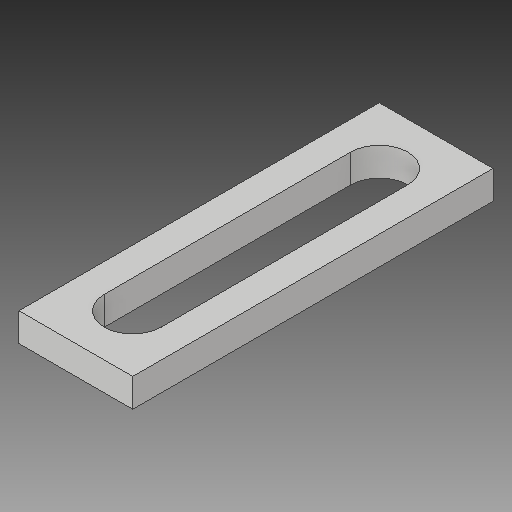
# Autodesk Inventor part: Marque
Saved by Autodesk Inventor 2017 (Build 210142000, 142)
## iProperties
Created: 2019-03-08
Part Number: Marque
Material: Generic
Document SubType Name: Modeling
Designer: Mitch
Density: 1 g/cm^3
Appearance: Default
Mass: 208.724 g
Surface Area: 425.806 cm^2
Volume: 208.724 cm^3
Author: Mitch
Autodesk Inventor part; units mm, degrees
ref_plane "YZ Plane" through (0, 0, 0) normal (1, 0, 0) x (0, 1, 0)
ref_plane "XZ Plane" through (0, 0, 0) normal (0, 1, 0) x (-1, 0, 0)
ref_plane "XY Plane" through (0, 0, 0) normal (0, 0, 1) x (1, 0, 0)
sketch "Sketch1" plane through (0, 0, 0) normal (0, 1, 0) x (-1, 0, 0)
  line L0 (0, 0) -> (76.2, 0)
  line L1 (76.2, 0) -> (76.2, -241.3)
  line L2 (76.2, -241.3) -> (0, -241.3)
  line L3 (0, -241.3) -> (0, 0)
  dimension "d0" = 76.2
  dimension "d1" = 241.3
  constraints: 8 end point, 2 parallel, 1 horizontal, 1 perpendicular
  measures "d0" distance of L1.end L2.end
  measures "d1" distance of L0.end L1.end
extrude "Extrusion1" add sketch "Sketch1" along normal blind 19.05
sketch "Sketch3" plane through (0, 19.05, 0) normal (0, 1, 0) x (1, 0, 0)
  line L0 (-76.2, 0) -> (0, 0) projected
  line L1 (0, 0) -> (0, 241.3) projected
  line L2 (0, 241.3) -> (-76.2, 241.3) projected
  line L3 (-76.2, 241.3) -> (-76.2, 0) projected
  line L4 (-38.1, 19.05) -> (-38.1, 19.05)
  line L5 (-19.05, 38.1) -> (-19.05, 203.2)
  line L6 (-38.1, 222.25) -> (-38.1, 222.25)
  line L7 (-57.15, 203.2) -> (-57.15, 38.1)
  arc A0 (-57.15, 38.1) -> (-38.1, 19.05) centre (-38.1, 38.1) ccw
  arc A1 (-38.1, 19.05) -> (-19.05, 38.1) centre (-38.1, 38.1) ccw
  arc A2 (-19.05, 203.2) -> (-38.1, 222.25) centre (-38.1, 203.2) ccw
  arc A3 (-38.1, 222.25) -> (-57.15, 203.2) centre (-38.1, 203.2) ccw
  dimension "d11" = 19.05
  dimension "d12" = 19.05
  constraints: 8 end point, 8 point on circle, 8 tangent, 4 centre point, 3 equal radius, 3 other
  measures "d11" distance between parallel lines of L3 L7
  measures "d12" radius of A0
extrude "Extrusion3" cut sketch "Sketch3" against normal blind 25.4 contours A1 A0 L7 A3 A2 L5
body "Solid1"
